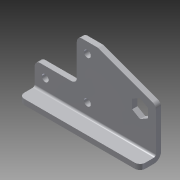
# Autodesk Inventor part: Spacer 3 (R-L)
Saved by Autodesk Inventor 2014 (Build 180170000, 170)
## iProperties
Created: 2014-01-17
Part Number: Spacer 3 (R-L)
Material: Aluminum 6061
Document SubType Name: Sheet Metal
Designer: Michael
Density: 2.71 g/cm^3
Sheet Metal Rule: Default
Appearance: Aluminum - Flat
Author: Michael
Autodesk Inventor part; units mm, degrees
ref_plane "YZ Plane" through (0, 0, 0) normal (1, 0, 0) x (0, 1, 0)
ref_plane "XZ Plane" through (0, 0, 0) normal (0, 1, 0) x (-1, 0, 0)
ref_plane "XY Plane" through (0, 0, 0) normal (0, 0, 1) x (1, 0, 0)
sketch "Sketch1" plane through (0, 0, 0) normal (0, 0, 1) x (1, 0, 0)
  line L0 (0, 0) -> (0, 12.7)
  line L1 (0, 12.7) -> (25.4, 12.7)
  line L2 (25.4, 12.7) -> (25.4, 38.1)
  line L3 (25.4, 38.1) -> (38.1, 38.1)
  line L4 (38.1, 38.1) -> (73.025, 25.4)
  line L5 (73.025, 25.4) -> (73.025, 0)
  line L6 (73.025, 0) -> (0, 0)
  line L7 (58.7375, 21.7996) -> (63.5, 24.5493)
  line L8 (63.5, 24.5493) -> (68.2625, 21.7996)
  line L9 (68.2625, 21.7996) -> (68.2625, 16.3004)
  line L10 (68.2625, 16.3004) -> (63.5, 13.5507)
  line L11 (63.5, 13.5507) -> (58.7375, 16.3004)
  line L12 (58.7375, 16.3004) -> (58.7375, 21.7996)
  circle A0 centre (6.35, 6.35) radius 2.0701
  circle A1 centre (31.75, 6.35) radius 2.0701
  circle A2 centre (31.75, 31.75) radius 2.0701
  point P0 (63.5, 19.05)
  dimension "d0" = 12.7
  dimension "d1" = 25.4
  dimension "d2" = 25.4
  dimension "d3" = 12.7
  dimension "d4" = 73.025
  dimension "d5" = 9.525
  dimension "d6" = 19.05
  dimension "d7" = 9.525
  dimension "d8" = 90
  dimension "d9" = 25.4
  dimension "d10" = 4.1402
  dimension "d11" = 6.35
  dimension "d12" = 6.35
  dimension "d15" = 25.4
  dimension "d22" = 25.4
  measures "d0" distance of L0.start L0.end
  measures "d1" distance of L0.end L1.end
  measures "d2" distance of L1.end L2.end
  measures "d3" distance of L2.end L3.end
  measures "d4" distance of L5.end L0.start
  measures "d5" distance between parallel lines of L12 L9
  measures "d6" distance from line of L6 point (63.5, 19.05)
  measures "d7" distance from line of L5 point (63.5, 19.05)
  measures "d8" angle of L6 L9
  measures "d9" distance of L4.end L5.end
  measures "d10" diameter of A0
  measures "d11" distance from line of L0 A0.centre
  measures "d12" distance from line of L1 A0.centre
  measures "d15" distance of A0.centre A1.centre
  measures "d22" distance of A1.centre A2.centre
extrude "Plate1" add sketch "Sketch1" along normal blind 3.175
sketch "Sketch2" plane through (73.025, -1.27, 4.445) normal (0, -1, 0) x (1, 0, 0)
  line L0 (-73.025, 0) -> (0, 0)
  line L1 (0, 0) -> (0, 8.255)
  line L2 (0, 8.255) -> (-73.025, 8.255)
  line L3 (-73.025, 8.255) -> (-73.025, 0)
  constraints: 6 end point, 1 horizontal, 1 perpendicular, 1 vertical
edge flange "Flange1" height 12.7 angle 90 thickness 3.175 bend radius 1.27 thickness toward (0, -1, 0) relief straight relief width 3.175 relief depth 1.5875 edges at (36.5125, 0, 3.175) wall of the first edge with corners at (0, -1.27, 4.445) (73.025, -1.27, 4.445) (73.025, -1.27, 12.7) (0, -1.27, 12.7)
bend "Bend1"
corner "Corner1"
fillet "Fillet2" radius 3.175 7 edges at (73.025, 25.4, 1.5875) (38.1, 38.1, 1.5875) (25.4, 38.1, 1.5875) (25.4, 12.7, 1.5875) (0, 12.7, 1.5875) (0, -2.8575, 12.7) (73.025, -2.8575, 12.7)
equation "\"d29\" = BendReliefWidth"
equation "\"d30\" = BendReliefDepth"
equation "\"d31\" = MinimumRemnant"
equation "\"d32\" = BendRadius"
equation "\"d36\" = CornerReliefSize"
equation "\"d37\" = GapSize"
equation "\"d38\" = JacobiRadiusSize"
equation "\"BendRadius\" = Thickness"
equation "\"BendReliefWidth\" = Thickness"
equation "\"BendReliefDepth\" = 0.5 * Thickness"
equation "\"CornerReliefSize\" = 4 * Thickness"
equation "\"MinimumRemnant\" = 2 * Thickness"
equation "\"TransitionRadius\" = BendRadius"
equation "\"JacobiRadiusSize\" = BendRadius"
equation "\"GapSize\" = Thickness"
equation "\"d27\" = BendRadius"
equation "\"Thickness\" = 3.175"
body "Solid1"
